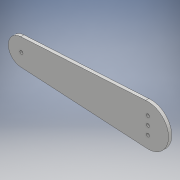
# Autodesk Inventor part: planos robot
Saved by Autodesk Inventor 2018 (Build 220112000, 112)
## iProperties
Created: 2020-03-10
Part Number: planos robot
Material: Genérico
Document SubType Name: Modeling
Designer: sala.ceri
Density: 1 g/cm^3
Appearance: Valor por defecto
Author: sala.ceri
Autodesk Inventor part; units mm, degrees
ref_plane "YZ Plane" through (0, 0, 0) normal (1, 0, 0) x (0, 1, 0)
ref_plane "XZ Plane" through (0, 0, 0) normal (0, 1, 0) x (-1, 0, 0)
ref_plane "XY Plane" through (0, 0, 0) normal (0, 0, 1) x (1, 0, 0)
sketch "Boceto1" plane through (0, 0, 0) normal (0, 1, 0) x (-1, 0, 0)
  arc A0 (120.2602, -12.5039) -> (120.7259, 12.475) centre (120.0354, -0.0059) ccw
  line L0 (2.2617, 19.3684) -> (120.7259, 12.475)
  line L1 (2.266, -19.3679) -> (119.9998, -12.5039)
  arc A1 (2.2617, 19.3684) -> (2.266, -19.3679) centre (0, 0) ccw
  circle A2 centre (120.0354, -0.0059) radius 1.5
  circle A3 centre (0, 0) radius 1.5
  circle A4 centre (0, -8) radius 1.5
  circle A5 centre (0, 8) radius 1.5
  line L2 (119.9998, -12.5039) -> (120.2602, -12.5039)
  dimension "d107" = 3
  constraints: 6 centre point, 6 end point, 4 point on circle, 2 coincident, 1 horizontal
  measures "d107" diameter of A2
extrude "Extrusión1" add sketch "Boceto1" along normal blind 3
